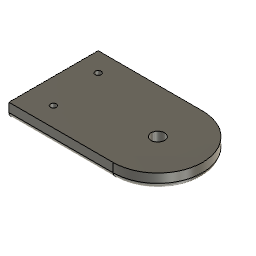
robosoc_body_holder_not_motor_side_V.1 (Autodesk Fusion 360 design; units mm, degrees)
part number: 2026-02-11-17-28-22-417
Autodesk Fusion 360 part; units mm, degrees
note: some values were not read from the file. Set by a fixed rule: the direction of a hole.
sketch "Sketch1" plane through (0, 0, 0) normal (0, 0, 1) x (1, 0, 0)
  line L0 (0, 0) -> (35, 0)
  line L1 (35, 30) -> (0, 30)
  line L2 (0, 30) -> (0, 0)
  circle A0 centre (35, 15) radius 2.25
  arc A1 (35, 0) -> (35, 30) centre (35, 15) ccw
  line L3 (15, 0) -> (15, 30)
  line L4 (15, 15) -> (0, 30) construction
  line L5 (7.5, 22.5) -> (7.5, 30) construction
  line L6 (7.5, 22.5) -> (0, 22.5) construction
  circle A2 centre (6.5, 23.5) radius 1
  circle A3 centre (8.5, 23.5) radius 1 construction
  circle A4 centre (8.5, 6.5) radius 1
  line L7 (15, 0) -> (0, 15) construction
  line L8 (7.5, 7.5) -> (7.5, 0) construction
  line L9 (7.5, 7.5) -> (15, 7.5) construction
  point P0 (40, 0)
  point P1 (15, 15)
  dimension "d1" = 30
  dimension "d7" = 35
  dimension "d8" = 35
  dimension "d9" = 4.5
  dimension "d14" = 2
  dimension "d36" = 2
  constraint horizontal L0
  constraint horizontal L1
  constraint vertical L2
  constraint coincident L0.start L2.end
  constraint coincident P0 L0
  constraint coincident A0.centre A1.centre
  constraint coincident L0 L3.start
  constraint coincident L1 L3.end
  constraint perpendicular L1 L3
  constraint midpoint L4 L5.start
  constraint coincident L1 L5.end
  constraint perpendicular L1 L5
  constraint coincident L2 L6.end
  constraint perpendicular L2 L6
  constraint coincident L4 A2.centre
  constraint tangent L5 A2
  constraint tangent L6 A2
  constraint symmetric L5 A2 A3
  constraint tangent L0 A1
  constraint midpoint L3 P1
  constraint coincident P1 L4.start
  constraint midpoint L2 L7.end
  constraint midpoint L7 L8.start
  constraint coincident L0 L8.end
  constraint perpendicular L0 L8
  constraint coincident L3 L9.end
  constraint perpendicular L3 L9
  constraint tangent A4 L9
  constraint tangent A4 L8
  measures "d1" distance of L0.start L1.end
  measures "d7" distance of L0.start L0.end
  measures "d8" distance of L1.end L1.start
  measures "d9" diameter of A0
  measures "d14" diameter of A2
  measures "d36" diameter of A4
extrude "Extrude1" add sketch "Sketch1" along normal blind 5 contours L0 L1 L2 L3 | L0 L1 A1 L3 | A0 | A2 | A4 makes body 1
hole "Hole1" at (8.5, 6.5, 0) at (6.5, 23.5, 0) direction (0, 0, 1) diameter 2 end through all counterbore diameter 2.3 counterbore depth 1 bodies 1
sketch "Sketch2" plane through (0, 0, 5) normal (0, 0, 1) x (-1, 0, 0)
  circle A0 centre (-8.5, -6.5) radius 1
  circle A1 centre (-6.5, -23.5) radius 1
  arc A2 (-35, 0) -> (-35, -30) centre (-35, -15) ccw
  line L0 (-35, -30) -> (0, -30)
  line L1 (0, -30) -> (0, 0)
  line L2 (0, 0) -> (-35, 0)
  circle A3 centre (-35, -15) radius 2.25
fillet "Fillet1" radius 2 3 edges at (17.5, 0, 0) (50, 15, 0) (17.5, 30, 0) on bodies 1
ref_plane "WorkPlane1" through (25, 15, 22.5) normal (0, 0, 1) x (1, 0, 0)
mirror "Mirror1" about plane through (25, 15, 22.5) normal (0, 0, 1) of bodies 1 makes body 2
extrude "Extrude2" cut sketch "Sketch2" against normal blind 4 contours A3 bodies 1
sketch "Sketch3" plane through (0, 0, 40) normal (0, 0, -1) x (1, 0, 0)
  circle A0 centre (8.5, -6.5) radius 1
  circle A1 centre (6.5, -23.5) radius 1
  arc A2 (35, -30) -> (35, 0) centre (35, -15) ccw
  line L0 (35, 0) -> (0, 0)
  line L1 (0, 0) -> (0, -30)
  line L2 (0, -30) -> (35, -30)
  line L3 (31.4, -14.9863) -> (24.6174, -26.7346)
  line L4 (35, -15) -> (24.8695, -28.0239) construction
  arc A3 (24.6174, -26.7346) -> (26.1812, -27.951) centre (25.4835, -27.2346) ccw
  line L5 (35.8992, -18.4859) -> (26.1812, -27.951)
  line L6 (31.4, -14.9863) -> (35.8992, -18.4859) construction
  arc A4 (35.8992, -18.4859) -> (31.4, -14.9863) centre (35, -15) ccw
  point P0 (35, -15)
  point P1 (35, -15)
  dimension "d30" = 2
  dimension "d31" = 5.7
  dimension "d32" = 16.5
  dimension "d33" = 7.2
  constraint coincident P1 P0
  constraint coincident L4.end A3
  constraint tangent A3 L5
  constraint tangent L3 A3
  constraint perpendicular L4 L6
  constraint coincident A3.centre L4
  measures "d30" diameter of A3
  measures "d31" distance of L3.start L5.start
  measures "d32" distance of L4.end P1
  measures "d33" diameter of A4
extrude "Extrude3" cut sketch "Sketch3" against normal blind 1.5 contours L3 A3 L5 A4 bodies 2
hidden bodies 2
equation "d1 = breadth"
equation "breadth = 30 mm"
equation "length = 50 mm"
equation "d6 = 15 mm"
equation "d7 = length - d6"
equation "d8 = d7"
equation "d27 = ( 35 / 2 ) * 1 mm"
equation "d36 = d14"
